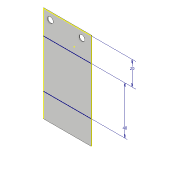
# Autodesk Inventor part: acrylic base
Saved by Autodesk Inventor 2019 (Build 230136000, 136)
## iProperties
Created: 2019-11-12
Part Number: acrylic base
Material: Generic
Document SubType Name: Sheet Metal
Designer: User
Density: 1 g/cm^3
Sheet Metal Rule: Default_mm
Appearance: Default
Author: User
Autodesk Inventor part; units mm, degrees
ref_plane "YZ Plane" through (0, 0, 0) normal (1, 0, 0) x (0, 1, 0)
ref_plane "XZ Plane" through (0, 0, 0) normal (0, 1, 0) x (-1, 0, 0)
ref_plane "XY Plane" through (0, 0, 0) normal (0, 0, 1) x (1, 0, 0)
sketch "Sketch1" plane through (0, 0, 0) normal (0, 0, 1) x (1, 0, 0)
  line L0 (-26.0465, 14.8837) -> (13.9535, 14.8837)
  line L1 (13.9535, 14.8837) -> (13.9535, -65.1163)
  line L2 (13.9535, -65.1163) -> (-26.0465, -65.1163)
  line L3 (-26.0465, -65.1163) -> (-26.0465, 14.8837)
  point P0 (0, 0)
  dimension "d0" = 40
  dimension "d1" = 80
  measures "d0" distance of L0.start L0.end
  measures "d1" distance of L0.end L1.end
extrude "Plate1" add sketch "Sketch1" along normal blind 0.5
sketch "Sketch6" plane through (0, 0, 0) normal (0, 0, -1) x (-1, 0, 0)
  point P0 (0, 0)
sketch "Sketch7" plane through (0, 0, 0.5) normal (0, 0, 1) x (1, 0, 0)
  line L0 (-26.0465, -65.1163) -> (-26.0465, 14.8837) projected
  line L1 (-26.0465, -5.1163) -> (13.9535, -5.1163)
  line L2 (13.9535, 14.8837) -> (13.9535, -65.1163) projected
  line L3 (-26.0465, -45.1163) -> (13.9535, -45.1163)
  line L4 (-26.0465, 14.8837) -> (13.9535, 14.8837) projected
  point P0 (0, 0)
  dimension "d10" = 20
  dimension "d11" = 40
  constraints: 4 end point, 2 horizontal, 2 point on line
  measures "d10" distance between parallel lines of L1 L4
  measures "d11" distance between parallel lines of L3 L1
sketch "Sketch10" plane through (0, 0, 0.5) normal (0, 0, 1) x (1, 0, 0)
  point P0 (0, 0)
  point P1 (-20.0888, 9.1588)
  point P2 (6.2939, 9.263)
hole "Hole3" at (-20.0888, 9.1588, 0.5) at (6.2939, 9.263, 0.5) direction (0, 0, -1) diameter 4.82 depth 0.5 tip angle 118
equation "\"d25\" = Thickness"
equation "\"d2\" = Thickness"
equation "\"BendRadius\" = Thickness"
equation "\"BendReliefWidth\" = Thickness"
equation "\"BendReliefDepth\" = 0.5 * Thickness"
equation "\"CornerReliefSize\" = 4 * Thickness"
equation "\"MinimumRemnant\" = 2 * Thickness"
equation "\"TransitionRadius\" = BendRadius"
equation "\"JacobiRadiusSize\" = BendRadius"
equation "\"GapSize\" = Thickness"
equation "\"Thickness\" = 0.5"
body "Solid1"
